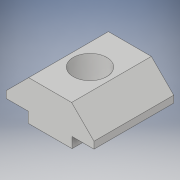
# Autodesk Inventor part: T-Brick
Saved by Autodesk Inventor 2019 (Build 230136000, 136)
## iProperties
Created: 2018-10-16
Part Number: T-Brick
Material: Generisch
Document SubType Name: Modeling
Designer: janbe
Density: 1 g/cm^3
Appearance: Vorgabe
Author: janbe
Autodesk Inventor part; units mm, degrees
ref_plane "YZ Plane" through (0, 0, 0) normal (1, 0, 0) x (0, 1, 0)
ref_plane "XZ Plane" through (0, 0, 0) normal (0, 1, 0) x (-1, 0, 0)
ref_plane "XY Plane" through (0, 0, 0) normal (0, 0, 1) x (1, 0, 0)
sketch "Skizze1" plane through (0, 0, 0) normal (0, 0, 1) x (1, 0, 0)
  line L0 (-2.7002, -2.1223) -> (-2.7002, -3.4436)
  line L1 (-5.4502, -2.1223) -> (-2.7002, -2.1223)
  line L2 (-5.4502, -1.2612) -> (-5.4502, -2.1223)
  line L3 (-2.6446, 1.5444) -> (-5.4502, -1.2612)
  line L4 (0.3248, 1.5444) -> (-2.6446, 1.5444)
  line L5 (2.7441, 1.5444) -> (0.3248, 1.5444)
  line L6 (5.5498, -1.2612) -> (2.7441, 1.5444)
  line L7 (5.5498, -2.1223) -> (5.5498, -1.2612)
  line L8 (2.7998, -2.1223) -> (5.5498, -2.1223)
  line L9 (2.7998, -3.4436) -> (2.7998, -2.1223)
  line L10 (-2.7002, -3.4436) -> (2.7998, -3.4436)
  point P0 (0, 0)
  dimension "d0" = 11
  dimension "d1" = 1.5444
  constraints: 22 end point, 2 horizontal
  measures "d0" distance between parallel lines of L7 L2
  measures "d1" distance from line of L4 point (0, 0)
extrude "Extrusion1" add sketch "Skizze1" along normal blind 10
sketch "Skizze2" plane through (-2.6446, 1.5444, 0) normal (0, 1, 0) x (1, 0, 0)
  line L0 (5.3888, 0) -> (0, 0) projected
  line L1 (0, 0) -> (0, -10) projected
  line L2 (5.3888, -10) -> (0, -10) projected
  line L3 (5.3888, 0) -> (5.3888, -10) projected
  circle A0 centre (2.6944, -5) radius 2.1
  point P0 (2.6446, 0)
  dimension "d4" = 4.2
  constraints: 1 centre point
  measures "d4" diameter of A0
extrude "Extrusion2" cut sketch "Skizze2" against normal up to surface (4.988 mm away) contours A0
